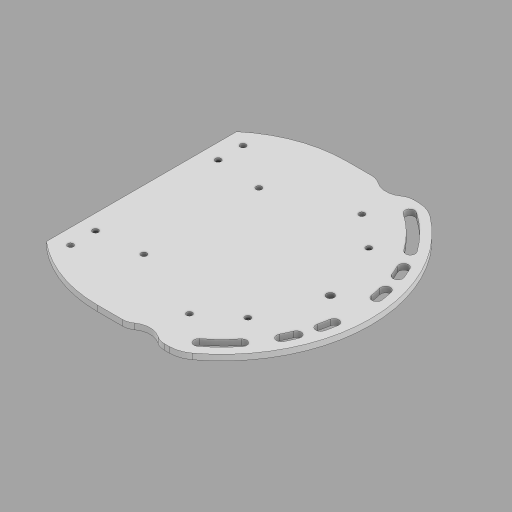
# Autodesk Inventor part: V_3
Saved by Autodesk Inventor 2024.2 (Build 282272000, 272)
## iProperties
Created: 2024-01-02
Part Number: V_3
Material: Типовые
Document SubType Name: Modeling
Designer: Fedor Orlov
Density: 1 g/cm^3
Appearance: По умолчанию
Author: Fedor Orlov
Autodesk Inventor part; units mm, degrees
ref_plane "YZ Plane" through (0, 0, 0) normal (1, 0, 0) x (0, 1, 0)
ref_plane "XZ Plane" through (0, 0, 0) normal (0, 1, 0) x (-1, 0, 0)
ref_plane "XY Plane" through (0, 0, 0) normal (0, 0, 1) x (1, 0, 0)
sketch "Эскиз1" plane through (0, 0, 0) normal (0, 1, 0) x (-1, 0, 0)
  arc A0 (42, 49.6085) -> (42, -49.6085) centre (0, 0) ccw
  line L0 (42, 49.6085) -> (42, -49.6085)
  arc A1 (42, -49.6085) -> (42, 49.6085) centre (0, 0) ccw construction
  line L1 (34, 55.3986) -> (34, -55.3986) construction
  circle A2 centre (34, 45) radius 1.5
  circle A3 centre (34, -45) radius 1.5
  line L2 (-28, 58.66) -> (-28, -58.66) construction
  line L3 (0, 0) -> (-28, -55) construction
  line L4 (0, 0) -> (-56.516, 0) construction
  circle A4 centre (-56.516, 0) radius 2
  circle A5 centre (-28, 45) radius 1.5
  circle A6 centre (-28, -45) radius 1.5
  dimension "d0" = 130
  dimension "d1" = 42
  dimension "d4" = 8
  dimension "d5" = 3
  dimension "d6" = 3
  dimension "d7" = 45
  dimension "d8" = 45
  dimension "d9" = 70
  dimension "d12" = 55
  dimension "d16" = 61.7171
  dimension "d18" = 4
  dimension "d20" = 3
  dimension "d21" = 45
  dimension "d22" = 3
  dimension "d38" = 56.516
  constraints: 10 end point, 8 point on circle, 7 centre point, 5 point on line, 3 vertical, 2 coincident, 1 horizontal
  measures "d0" diameter of A0
  measures "d1" distance from line of point (0, 0) L0
  measures "d4" distance between parallel lines of L0 L1
  measures "d5" diameter of A2
  measures "d6" diameter of A3
  measures "d7" vertical distance of point (0, 0) A3.centre
  measures "d8" vertical distance of A2.centre point (0, 0)
  measures "d9" distance between parallel lines of L0 L2
  measures "d12" vertical distance of point (0, 0) L3.end
  measures "d16" distance of L3.start L3.end
  measures "d18" diameter of A4
  measures "d20" diameter of A5
  measures "d21" vertical distance of A5.centre point (0, 0)
  measures "d22" diameter of A6
  measures "d38" distance of L4.end point (0, 0)
extrude "Выдавливание1" add sketch "Эскиз1" along normal blind 3
sketch "Эскиз2" plane through (0, 3, 0) normal (0, 1, 0) x (1, 0, 0)
  circle A0 centre (-34, -45) radius 1.5 projected
  circle A1 centre (-34, 45) radius 1.5 projected
  line L0 (-34, -45) -> (-34, 45) construction
  circle A2 centre (0, 0) radius 55 construction
  line L1 (0, 0) -> (0, -55) construction
  line L2 (0, 0) -> (45.0534, -31.5467) construction
  circle A3 centre (45.0534, -31.5467) radius 1.5
  circle A4 centre (56.516, 0) radius 2 projected
  line L3 (0, 0) -> (56.516, 0) construction
  circle A5 centre (45.0534, 31.5467) radius 1.5
  circle A6 centre (-34, -32) radius 1.5
  circle A7 centre (-34, 32) radius 1.5
  line L4 (-42, 49.6085) -> (-42, -49.6085) projected
  point P0 (-42, 0)
  point P1 (-34, 0)
  dimension "d25" = 110
  dimension "d26" = 55
  dimension "d28" = 3
  dimension "d34" = 3
  dimension "d35" = 3
  dimension "d36" = 32
  dimension "d37" = 32
  constraints: 8 end point, 5 centre point, 2 coincident, 2 midpoint, 2 point on circle, 2 point on line, 2 vertical, 1 horizontal, 1 symmetric about line, 1 other
  measures "d25" diameter of A2
  measures "d26" angle of L1 L2
  measures "d28" diameter of A3
  measures "d34" diameter of A6
  measures "d35" diameter of A7
  measures "d36" vertical distance of point (-42, 0) A6.centre
  measures "d37" distance of A7.centre point (-34, 0)
extrude "Выдавливание2" cut sketch "Эскиз2" against normal blind 10 contours A3 | A5 | A6 | A7
chamfer "Фаска1" distance 1.6 angle 45 4 edges at (43.5534, 0, 31.5467) (43.5534, 0, -31.5467) (-35.5, 0, -32) (-35.5, 0, 32)
sketch "Эскиз3" plane through (0, 3, 0) normal (0, 1, 0) x (1, 0, 0)
  circle A0 centre (-34, -45) radius 1.5 projected
  circle A1 centre (-34, 45) radius 1.5 projected
  line L0 (-34, -45) -> (-34, 45) construction
  line L1 (-34, 45) -> (12.5, 45) construction
  line L2 (-10.75, 45) -> (-10.75, -55.9117) construction
  circle A2 centre (-10.75, -30) radius 1.5
  circle A3 centre (-10.75, 30) radius 1.5
  point P0 (0, 0)
  dimension "d39" = 46.5
  dimension "d40" = 3
  dimension "d41" = 3
  dimension "d42" = 30
  dimension "d43" = 30
  constraints: 6 end point, 2 centre point, 2 point on line, 2 vertical, 1 midpoint, 1 perpendicular
  measures "d39" distance of L0.end L1.end
  measures "d40" diameter of A2
  measures "d41" diameter of A3
  measures "d42" vertical distance of point (0, 0) A2.centre
  measures "d43" vertical distance of point (0, 0) A3.centre
extrude "Выдавливание3" cut sketch "Эскиз3" against normal blind 10 contours A2 | A3
sketch "Эскиз4" plane through (0, 3, 0) normal (0, 1, 0) x (1, 0, 0)
  arc A0 (42.2049, -65) -> (42.2049, 65) centre (0, 0) ccw
  arc A1 (-42, -49.6085) -> (-42, 49.6085) centre (0, 0) ccw projected
  line L0 (0, -65) -> (42.2049, -65)
  line L1 (0, 65) -> (42.2049, 65)
  arc A2 (42.2049, 65) -> (42.2049, -65) centre (0, 0) ccw construction
  line L2 (0, 0) -> (65, 0) construction
  line L3 (0, 0) -> (75.9442, -15.451) construction
  line L4 (0, 0) -> (70.522, -32.1387) construction
  line L5 (0, 0) -> (54.3205, -55.2769) construction
  line L6 (0, 0) -> (57.5937, 51.8576) construction
  line L7 (0, 0) -> (41.0687, 65.7237) construction
  circle A3 centre (0, 0) radius 70.5 construction
  arc A4 (43.3889, -55.5666) -> (54.8009, -44.3521) centre (0, 0) ccw construction
  arc A5 (44.9275, -57.5371) -> (56.7442, -45.9249) centre (0, 0) ccw
  arc A6 (41.8503, -53.5962) -> (52.8576, -42.7793) centre (0, 0) ccw
  arc A7 (41.8503, -53.5962) -> (44.9275, -57.5371) centre (43.3889, -55.5666) ccw
  arc A8 (56.7442, -45.9249) -> (52.8576, -42.7793) centre (54.8009, -44.3521) ccw
  arc A9 (62.8501, -31.9393) -> (65.3382, -26.4795) centre (0, 0) ccw construction
  arc A10 (65.0788, -33.0719) -> (67.6552, -27.4185) centre (0, 0) ccw
  arc A11 (60.6214, -30.8067) -> (63.0213, -25.5405) centre (0, 0) ccw
  arc A12 (60.6214, -30.8067) -> (65.0788, -33.0719) centre (62.8501, -31.9393) ccw
  arc A13 (67.6552, -27.4185) -> (63.0213, -25.5405) centre (65.3382, -26.4795) ccw
  arc A14 (68.424, -16.9825) -> (69.6202, -11.1029) centre (0, 0) ccw construction
  arc A15 (70.8504, -17.5847) -> (72.089, -11.4967) centre (0, 0) ccw
  arc A16 (65.9976, -16.3803) -> (67.1514, -10.7092) centre (0, 0) ccw
  arc A17 (65.9976, -16.3803) -> (70.8504, -17.5847) centre (68.424, -16.9825) ccw
  arc A18 (72.089, -11.4967) -> (67.1514, -10.7092) centre (69.6202, -11.1029) ccw
  arc A19 (57.4063, 40.9238) -> (39.8696, 58.1435) centre (0, 0) ccw construction
  arc A20 (59.442, 42.375) -> (41.2834, 60.2053) centre (0, 0) ccw
  arc A21 (55.3707, 39.4726) -> (38.4558, 56.0817) centre (0, 0) ccw
  arc A22 (55.3707, 39.4726) -> (59.442, 42.375) centre (57.4063, 40.9238) ccw
  arc A23 (41.2834, 60.2053) -> (38.4558, 56.0817) centre (39.8696, 58.1435) ccw
  line L8 (0, 0) -> (75.9442, 15.451) construction
  line L9 (0, 0) -> (70.522, 32.1387) construction
  arc A24 (65.3382, 26.4795) -> (62.8501, 31.9393) centre (0, 0) ccw construction
  arc A25 (67.6552, 27.4185) -> (65.0788, 33.0719) centre (0, 0) ccw
  arc A26 (63.0213, 25.5405) -> (60.6214, 30.8067) centre (0, 0) ccw
  arc A27 (65.0788, 33.0719) -> (60.6214, 30.8067) centre (62.8501, 31.9393) ccw
  arc A28 (63.0213, 25.5405) -> (67.6552, 27.4185) centre (65.3382, 26.4795) ccw
  arc A29 (69.6202, 11.1029) -> (68.424, 16.9825) centre (0, 0) ccw construction
  arc A30 (72.089, 11.4967) -> (70.8504, 17.5847) centre (0, 0) ccw
  arc A31 (67.1514, 10.7092) -> (65.9976, 16.3803) centre (0, 0) ccw
  arc A32 (70.8504, 17.5847) -> (65.9976, 16.3803) centre (68.424, 16.9825) ccw
  arc A33 (67.1514, 10.7092) -> (72.089, 11.4967) centre (69.6202, 11.1029) ccw
  point P0 (21.1024, -65)
  dimension "d46" = 155
  dimension "d53" = 11.5
  dimension "d54" = 24.5
  dimension "d55" = 45.5
  dimension "d56" = 42
  dimension "d57" = 58
  dimension "d58" = 65
  dimension "d60" = 65
  dimension "d61" = 141
  dimension "d62" = 5
  dimension "d63" = 5
  dimension "d64" = 5
  dimension "d65" = 8
  dimension "d66" = 3
  dimension "d67" = 3
  dimension "d68" = 3
  dimension "d69" = 3
  dimension "d70" = 2.5
  dimension "d71" = 8
  dimension "d72" = 8
  dimension "d73" = 3
  constraints: 76 point on circle, 33 centre point, 20 end point, 16 tangent, 14 symmetric about line, 7 coincident, 4 concentric, 2 horizontal, 1 midpoint, 1 parallel, 10 other
  measures "d46" diameter of A0
  measures "d53" angle of L2 L3
  measures "d54" angle of L2 L4
  measures "d55" angle of L2 L5
  measures "d56" angle of L6 L2
  measures "d57" angle of L2 L7
  measures "d58" distance from line of L0 point (0, 0)
  measures "d60" distance between parallel lines of L1 L2
  measures "d61" diameter of A3
  measures "d62" diameter of A12
  measures "d63" diameter of A18
  measures "d64" diameter of A22
  measures "d65" distance from line of L6 A19.start
  measures "d66" distance from line of A14.end L3
  measures "d67" distance from line of A14.start L3
  measures "d68" distance from line of A3.end L4
  measures "d69" distance from line of A9.start L4
  measures "d70" radius of A8
  measures "d71" distance from line of A4.end L5
  measures "d72" distance from line of A3.start L5
  measures "d73" distance from line of A19.end L7
extrude "Выдавливание4" add sketch "Эскиз4" against normal blind 3
fillet "Сопряжение2" radius 15 2 edges at (42.2049, 1.5, 65) (42.2049, 1.5, -65)
sketch "Эскиз5" plane through (0, 3, 0) normal (0, 1, 0) x (1, 0, 0)
  line L0 (24, -72) -> (24, 72) construction
  arc A0 (41.8503, -53.5962) -> (52.8576, -42.7793) centre (0, 0) ccw projected
  arc A1 (56.7442, -45.9249) -> (52.8576, -42.7793) centre (54.8009, -44.3521) ccw projected
  arc A2 (44.9275, -57.5371) -> (56.7442, -45.9249) centre (0, 0) ccw projected
  arc A3 (41.8503, -53.5962) -> (44.9275, -57.5371) centre (43.3889, -55.5666) ccw projected
  arc A4 (60.6214, -30.8067) -> (63.0213, -25.5405) centre (0, 0) ccw projected
  arc A5 (67.6552, -27.4185) -> (63.0213, -25.5405) centre (65.3382, -26.4795) ccw projected
  arc A6 (65.0788, -33.0719) -> (67.6552, -27.4185) centre (0, 0) ccw projected
  arc A7 (60.6214, -30.8067) -> (65.0788, -33.0719) centre (62.8501, -31.9393) ccw projected
  arc A8 (65.9976, -16.3803) -> (67.1514, -10.7092) centre (0, 0) ccw projected
  arc A9 (72.089, -11.4967) -> (67.1514, -10.7092) centre (69.6202, -11.1029) ccw projected
  arc A10 (70.8504, -17.5847) -> (72.089, -11.4967) centre (0, 0) ccw projected
  arc A11 (65.9976, -16.3803) -> (70.8504, -17.5847) centre (68.424, -16.9825) ccw projected
  arc A12 (55.3707, 39.4726) -> (38.4558, 56.0817) centre (0, 0) ccw projected
  arc A13 (41.2834, 60.2053) -> (38.4558, 56.0817) centre (39.8696, 58.1435) ccw projected
  arc A14 (59.442, 42.375) -> (41.2834, 60.2053) centre (0, 0) ccw projected
  arc A15 (55.3707, 39.4726) -> (59.442, 42.375) centre (57.4063, 40.9238) ccw projected
  arc A16 (67.1514, 10.7092) -> (65.9976, 16.3803) centre (0, 0) ccw projected
  arc A17 (70.8504, 17.5847) -> (65.9976, 16.3803) centre (68.424, 16.9825) ccw projected
  arc A18 (72.089, 11.4967) -> (70.8504, 17.5847) centre (0, 0) ccw projected
  arc A19 (67.1514, 10.7092) -> (72.089, 11.4967) centre (69.6202, 11.1029) ccw projected
  arc A20 (63.0213, 25.5405) -> (67.6552, 27.4185) centre (65.3382, 26.4795) ccw projected
  arc A21 (63.0213, 25.5405) -> (60.6214, 30.8067) centre (0, 0) ccw projected
  arc A22 (65.0788, 33.0719) -> (60.6214, 30.8067) centre (62.8501, 31.9393) ccw projected
  arc A23 (67.6552, 27.4185) -> (65.0788, 33.0719) centre (0, 0) ccw projected
  circle A24 centre (-10.75, 30) radius 1.5 projected
  circle A25 centre (-10.75, -30) radius 1.5 projected
  circle A26 centre (45.0534, 31.5467) radius 1.5 projected
  circle A27 centre (-34, 32) radius 1.5 projected
  circle A28 centre (45.0534, -31.5467) radius 1.5 projected
  circle A29 centre (-34, -32) radius 1.5 projected
  arc A30 (46.5, 62) -> (37.5, 65) centre (37.5, 50) ccw projected
  line L1 (37.5, 65) -> (0, 65) projected
  arc A31 (0, 65) -> (-42, 49.6085) centre (0, 0) ccw projected
  line L2 (-42, 49.6085) -> (-42, -49.6085) projected
  arc A32 (-42, -49.6085) -> (0, -65) centre (0, 0) ccw projected
  line L3 (0, -65) -> (37.5, -65) projected
  arc A33 (37.5, -65) -> (46.5, -62) centre (37.5, -50) ccw projected
  arc A34 (46.5, -62) -> (46.5, 62) centre (0, 0) ccw projected
  circle A35 centre (28, 45) radius 1.5 projected
  circle A36 centre (28, -45) radius 1.5 projected
  circle A37 centre (56.516, 0) radius 2 projected
  circle A38 centre (-34, 45) radius 1.5 projected
  circle A39 centre (-34, -45) radius 1.5 projected
  arc A40 (46.5, -62) -> (46.5, 62) centre (0, 0) ccw projected
  arc A41 (-42, -49.6085) -> (0, -65) centre (0, 0) ccw projected
  circle A42 centre (24, -72) radius 10.5
  circle A43 centre (24, 72) radius 10.5
  dimension "d74" = 72
  dimension "d75" = 72
  dimension "d76" = 32.516
  dimension "d77" = 21
  dimension "d78" = 21
  constraints: 2 centre point, 2 coincident, 2 end point, 1 vertical
  measures "d74" vertical distance of A37.centre L0.start
  measures "d75" vertical distance of A37.centre L0.end
  measures "d76" distance from line of L0 A37.centre
  measures "d77" diameter of A42
  measures "d78" diameter of A43
extrude "Выдавливание5" cut sketch "Эскиз5" against normal blind 3 contours A43 L1 | L1 A43 | A42 L3 | L3 A42
fillet "Сопряжение3" radius 8 4 edges at (31.8262, 1.5, 65) (16.1738, 1.5, 65) (16.1738, 1.5, -65) (31.8262, 1.5, -65)
equation "\"d60\" = d58"
equation "\"d67\" = d66"
